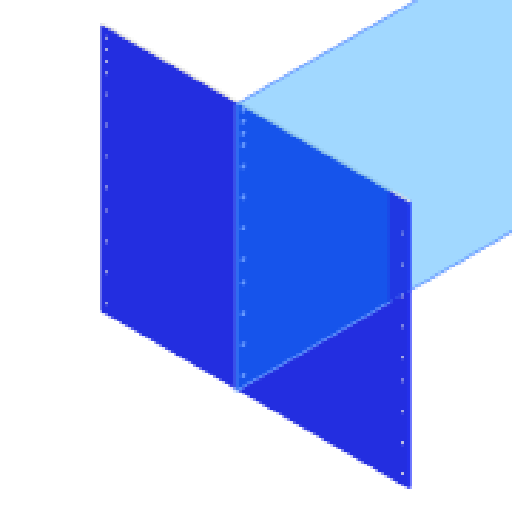
# Autodesk Inventor part: Боковая часть корпуса
Saved by Autodesk Inventor 2023.2 (Build 272271030, 271C)
## iProperties
Created: 2025-04-24
Part Number: Боковая часть корпуса
Material: Типовые
Document SubType Name: Modeling
Designer: Коноваленко
Density: 1 g/cm^3
Appearance: По умолчанию
Author: Коноваленко
Autodesk Inventor part; units mm, degrees
ref_plane "YZ Plane" through (0, 0, 0) normal (1, 0, 0) x (0, 1, 0)
ref_plane "XZ Plane" through (0, 0, 0) normal (0, 1, 0) x (-1, 0, 0)
ref_plane "XY Plane" through (0, 0, 0) normal (0, 0, 1) x (1, 0, 0)
sketch "Эскиз1" plane through (0, 0, 0) normal (0, 0, 1) x (1, 0, 0)
  line L0 (230, 185) -> (230, -185)
  line L1 (230, -185) -> (-230, -185)
  line L2 (-230, -185) -> (-230, 185)
  line L3 (-230, 185) -> (230, -185) construction
  line L4 (230, 185) -> (-230, -185) construction
  line L5 (-322, 0) -> (322, 0) construction
  line L6 (0, 259) -> (0, -259) construction
  line L7 (-230, 185) -> (230, 185)
  point P0 (0, 0)
  dimension "d2" = 370
  dimension "d4" = 460
  constraints: 12 end point, 3 perpendicular, 2 midpoint, 1 horizontal
  measures "d2" distance of L1.end L2.end
  measures "d4" distance of L0.end L1.end
extrude "Выдавливание1" add sketch "Эскиз1" along normal mid plane 4
sketch "Эскиз2" plane through (0, 0, 2) normal (0, 0, 1) x (1, 0, 0)
  circle A0 centre (-220, 172.5) radius 2 projected
  circle A1 centre (-220, 157.5) radius 2 projected
  circle A2 centre (-220, 142.5) radius 2 projected
  circle A3 centre (-220, 127.5) radius 2 projected
  circle A4 centre (-220, 100) radius 2 projected
  circle A5 centre (-220, 60) radius 2 projected
  circle A6 centre (-220, 20) radius 2 projected
  circle A7 centre (-220, -20) radius 2 projected
  circle A8 centre (-220, -50) radius 2 projected
  circle A9 centre (-220, -90) radius 2 projected
  circle A10 centre (-220, -130) radius 2 projected
  circle A11 centre (-220, -170) radius 2 projected
  circle A12 centre (220, 140) radius 2 projected
  circle A13 centre (220, 100) radius 2 projected
  circle A14 centre (220, 60) radius 2 projected
  circle A15 centre (220, 20) radius 2 projected
  circle A16 centre (220, -20) radius 2 projected
  circle A17 centre (220, -50) radius 2 projected
  circle A18 centre (220, -90) radius 2 projected
  circle A19 centre (220, -130) radius 2 projected
  circle A20 centre (220, -170) radius 2 projected
  point P0 (0, 0)
extrude "Выдавливание2" cut sketch "Эскиз2" against normal up to surface (4 mm away)
